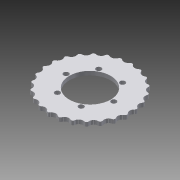
# Autodesk Inventor part: Small Sprocket
Saved by Autodesk Inventor 2015 (Build 190159000, 159)
## iProperties
Created: 2015-02-07
Part Number: Small Sprocket
Material: Aluminum 6061
Document SubType Name: Modeling
Designer: pltwe4
Density: 2.7 g/cm^3
Appearance: Aluminum - Flat
Author: pltwe4
Autodesk Inventor part; units mm, degrees
ref_plane "YZ Plane" through (0, 0, 0) normal (1, 0, 0) x (0, 1, 0)
ref_plane "XZ Plane" through (0, 0, 0) normal (0, 1, 0) x (-1, 0, 0)
ref_plane "XY Plane" through (0, 0, 0) normal (0, 0, 1) x (1, 0, 0)
sketch "Sketch1" plane through (0, 0, 0) normal (0, 1, 0) x (-1, 0, 0)
  circle A0 centre (0, 0) radius 42.1386
  circle A1 centre (0, 0) radius 39.5986 construction
  circle A2 centre (0, 0) radius 20.6375
  circle A3 centre (0, 0) radius 23.8125 construction
  circle A4 centre (23.8125, 0) radius 2.6162
  line L0 (0, -58.99404) -> (0, 58.99404) construction
  line L1 (-58.99404, 0) -> (58.99404, 0) construction
  circle A5 centre (11.90625, 20.62223) radius 2.6162
  circle A6 centre (-11.90625, 20.62223) radius 2.6162
  circle A7 centre (-23.8125, 0) radius 2.6162
  circle A8 centre (-11.90625, -20.62223) radius 2.6162
  circle A9 centre (11.90625, -20.62223) radius 2.6162
  line L2 (0, 0) -> (42.1386, 0) construction
  line L3 (0, 0) -> (40.914129, 10.084427) construction
  line L4 (0, 0) -> (37.311877, 19.582784) construction
  line L5 (0, 0) -> (31.541195, 27.94306) construction
  line L6 (0, 0) -> (23.937453, 34.679388) construction
  line L7 (0, 0) -> (14.942553, 39.400275) construction
  line L8 (0, 0) -> (5.079247, 41.831362) construction
  line L9 (0, 0) -> (-5.079247, 41.831362) construction
  line L10 (0, 0) -> (-14.942553, 39.400275) construction
  line L11 (0, 0) -> (-23.937453, 34.679388) construction
  line L12 (0, 0) -> (-31.541195, 27.94306) construction
  line L13 (0, 0) -> (-37.311877, 19.582784) construction
  line L14 (0, 0) -> (-40.914129, 10.084427) construction
  line L15 (0, 0) -> (-42.1386, 0) construction
  line L16 (0, 0) -> (-40.914129, -10.084427) construction
  line L17 (0, 0) -> (-37.311877, -19.582784) construction
  line L18 (0, 0) -> (-31.541195, -27.94306) construction
  line L19 (0, 0) -> (-23.937453, -34.679388) construction
  line L20 (0, 0) -> (-14.942553, -39.400275) construction
  line L21 (0, 0) -> (-5.079247, -41.831362) construction
  line L22 (0, 0) -> (5.079247, -41.831362) construction
  line L23 (0, 0) -> (14.942553, -39.400275) construction
  line L24 (0, 0) -> (23.937453, -34.679388) construction
  line L25 (0, 0) -> (31.541195, -27.94306) construction
  line L26 (0, 0) -> (37.311877, -19.582784) construction
  line L27 (0, 0) -> (40.914129, -10.084427) construction
  dimension "d0" = 84.2772
  dimension "d3" = 47.625
  dimension "d1" = 79.1972
  dimension "d2" = 41.275
  dimension "d4" = 5.2324
  dimension "d7" = 360
  dimension "d11" = 360
  constraints: 52 end point, 8 centre point, 4 coincident, 2 horizontal alignment, 2 point on line, 96 other
  measures "d1" diameter of A1
  measures "d2" diameter of A2
  measures "d4" diameter of A4
extrude "Extrusion1" add sketch "Sketch1" along normal blind 3.9624
sketch "Sketch2" plane through (0, 3.9624, 0) normal (0, 1, 0) x (1, 0, 0)
  circle A0 centre (0, 0) radius 20.6375
  circle A1 centre (-11.90625, 20.62223) radius 2.6162
  circle A2 centre (11.90625, 20.62223) radius 2.6162
  circle A3 centre (23.8125, 0) radius 2.6162
  circle A4 centre (11.90625, -20.62223) radius 2.6162
  circle A5 centre (-11.90625, -20.62223) radius 2.6162
  circle A6 centre (-23.8125, 0) radius 2.6162
  circle A7 centre (0, 0) radius 42.1386
  circle A8 centre (0, 0) radius 39.5986
  circle A9 centre (0, 0) radius 42.1386 construction
  line L0 (0, 0) -> (0, 42.1386) construction
  line L1 (0, 0) -> (-10.084427, 40.914129) construction
  line L2 (0, 0) -> (-19.582784, 37.311877) construction
  line L3 (0, 0) -> (-27.94306, 31.541195) construction
  line L4 (0, 0) -> (-34.679388, 23.937453) construction
  line L5 (0, 0) -> (-39.400275, 14.942553) construction
  line L6 (0, 0) -> (-41.831362, 5.079247) construction
  line L7 (0, 0) -> (-41.831362, -5.079247) construction
  line L8 (0, 0) -> (-39.400275, -14.942553) construction
  line L9 (0, 0) -> (-34.679388, -23.937453) construction
  line L10 (0, 0) -> (-27.94306, -31.541195) construction
  line L11 (0, 0) -> (-19.582784, -37.311877) construction
  line L12 (0, 0) -> (-10.084427, -40.914129) construction
  line L13 (0, 0) -> (0, -42.1386) construction
  line L14 (0, 0) -> (10.084427, -40.914129) construction
  line L15 (0, 0) -> (19.582784, -37.311877) construction
  line L16 (0, 0) -> (27.94306, -31.541195) construction
  line L17 (0, 0) -> (34.679388, -23.937453) construction
  line L18 (0, 0) -> (39.400275, -14.942553) construction
  line L19 (0, 0) -> (41.831362, -5.079247) construction
  line L20 (0, 0) -> (41.831362, 5.079247) construction
  line L21 (0, 0) -> (39.400275, 14.942553) construction
  line L22 (0, 0) -> (34.679388, 23.937453) construction
  line L23 (0, 0) -> (27.94306, 31.541195) construction
  line L24 (0, 0) -> (19.582784, 37.311877) construction
  line L25 (0, 0) -> (10.084427, 40.914129) construction
  line L26 (65.278771, 0) -> (-65.608839, 0) construction
  line L27 (0, 0) -> (5.079247, 41.831362) construction
  arc A10 (1.591047, 41.281262) -> (0, 42.1386) centre (0, 40.2336) ccw
  arc A11 (10.084427, 40.914129) -> (8.334439, 40.462466) centre (9.628531, 39.064485) ccw
  arc A12 (1.591047, 41.281262) -> (8.334439, 40.462466) centre (5.309777, 43.729946) ccw
  circle A13 centre (0, 0) radius 42.1386 construction
  arc A14 (-10.084427, 40.914129) -> (19.582784, 37.311877) centre (0, 0) ccw
  arc A15 (10.084427, 40.914129) -> (0, 42.1386) centre (0, 0) ccw
  dimension "d15" = 79.1972
  dimension "d20" = 3.81
  constraints: 54 end point, 15 point on circle, 6 centre point, 3 point on line, 3 tangent, 2 coincident, 1 equal radius, 1 perpendicular, 83 other
  measures "d15" diameter of A8
  measures "d20" diameter of A10
extrude "Extrusion2" cut sketch "Sketch2" against normal up to next contours A11 A12 A10 A7 picked at (4.974446, 40.968252)
pattern_circular "Circular Pattern1" count 26 over 360 about axis through (0, 0, 0) along (0, 1, 0) of "Extrusion2"
body "Solid1"
